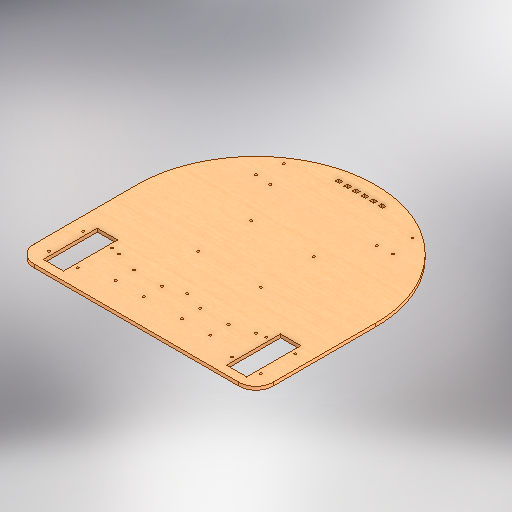
# Autodesk Inventor part: layer1
Saved by Autodesk Inventor 2026 (Build 300175050, 175E)
## iProperties
Created: 2025-06-04
Part Number: layer1
Material: Generic
Document SubType Name: Modeling
Designer: satom
Density: 1 g/cm^3
Appearance: Cherry - Natural Low Gloss
Author: satom
Autodesk Inventor part; units mm, degrees
ref_plane "YZ Plane" through (0, 0, 0) normal (1, 0, 0) x (0, 1, 0)
ref_plane "XZ Plane" through (0, 0, 0) normal (0, 1, 0) x (-1, 0, 0)
ref_plane "XY Plane" through (0, 0, 0) normal (0, 0, 1) x (1, 0, 0)
sketch "Sketch1" plane through (0, 0, 0) normal (0, 1, 0) x (-1, 0, 0)
  arc A0 (-177, 0) -> (177, 0) centre (0, 0) ccw
  line L0 (-177, 0) -> (-177, 151.6)
  line L1 (-151.6, 177) -> (151.6, 177)
  line L2 (177, 151.6) -> (177, 0)
  arc A1 (-151.6, 177) -> (-177, 151.6) centre (-151.6, 151.6) ccw
  arc A2 (177, 151.6) -> (151.6, 177) centre (151.6, 151.6) ccw
  point P0 (-177, 177)
  point P1 (177, 177)
  dimension "d0" = 354
  dimension "d98" = 177
  dimension "d99" = 177
  dimension "d101" = 354
  dimension "d102" = 177
  dimension "d217" = 25.4
  constraints: 6 end point, 6 point on circle, 4 point on line, 4 tangent, 3 centre point, 1 coincident, 1 equal radius, 1 parallel
  measures "d0" diameter of A0
  measures "d98" distance of point (177, 177) L2.end
  measures "d99" distance of L0.start point (-177, 177)
  measures "d101" distance between parallel lines of L0 L2
  measures "d102" distance from line of point (0, 0) L1
  measures "d217" radius of A1
extrude "Extrusion1" add sketch "Sketch1" along normal blind 5
sketch "Sketch8" plane through (0, 5, 0) normal (0, 1, 0) x (1, 0, 0)
  circle A0 centre (101.6, -101.6) radius 1.7
  circle A1 centre (101.6, 101.6) radius 1.7
  circle A2 centre (-101.6, 101.6) radius 1.7
  circle A3 centre (-101.6, -101.6) radius 1.7
  arc A4 (177, 0) -> (-177, 0) centre (0, 0) ccw construction
  line L0 (0, 177) -> (0, -177) construction
  line L1 (-151.6, -177) -> (151.6, -177) construction
  line L2 (-177, 0) -> (-177, -151.6) construction
  line L3 (177, -151.6) -> (177, 0) construction
  line L4 (-177, 0) -> (177, 0) construction
  circle A5 centre (0, -101.6) radius 1.7
  point P0 (0, 0)
  point P1 (-177, -177)
  point P2 (177, -177)
  dimension "d103" = 3.4
  dimension "d104" = 3.4
  dimension "d105" = 3.4
  dimension "d106" = 3.4
  dimension "d115" = 101.6
  dimension "d116" = 101.6
  dimension "d117" = 101.6
  dimension "d118" = 101.6
  dimension "d119" = 101.6
  dimension "d120" = 101.6
  dimension "d121" = 101.6
  dimension "d122" = 101.6
  dimension "d255" = 3.4
  dimension "d256" = 101.6
  constraints: 5 centre point, 4 end point, 2 coincident, 1 horizontal, 1 midpoint, 1 point on circle, 1 point on line
  measures "d103" diameter of A3
  measures "d104" diameter of A2
  measures "d105" diameter of A0
  measures "d106" diameter of A1
  measures "d115" distance from line of L4 A3.centre
  measures "d116" distance from line of L4 A2.centre
  measures "d117" distance from line of L4 A1.centre
  measures "d118" distance from line of L4 A0.centre
  measures "d119" distance from line of A0.centre L0
  measures "d120" distance from line of A3.centre L0
  measures "d121" distance from line of L0 A2.centre
  measures "d122" distance from line of A1.centre L0
  measures "d255" diameter of A5
  measures "d256" distance from line of L4 A5.centre
extrude "Stand-Offs" cut sketch "Sketch8" against normal through all
sketch "Sketch9" plane through (0, 5, 0) normal (0, 1, 0) x (1, 0, 0)
  line L0 (-150.65, -84.3) -> (-150.65, -164.3)
  line L1 (-150.65, -164.3) -> (-120.65, -164.3)
  line L2 (-120.65, -164.3) -> (-120.65, -84.3)
  line L3 (-120.65, -84.3) -> (-150.65, -84.3)
  circle A0 centre (-114.3, -98.9) radius 1.7
  circle A1 centre (-114.3, -149.7) radius 1.7
  circle A2 centre (-157, -149.7) radius 1.7
  circle A3 centre (-157, -98.9) radius 1.7
  arc A4 (177, 0) -> (-177, 0) centre (0, 0) ccw construction
  line L4 (0, 177) -> (0, -177) construction
  line L5 (-151.6, -177) -> (151.6, -177) construction
  line L6 (-120.65, -124.3) -> (-150.65, -124.3) construction
  line L7 (150.65, -164.3) -> (120.65, -164.3)
  line L8 (120.65, -164.3) -> (120.65, -84.3)
  line L9 (120.65, -84.3) -> (150.65, -84.3)
  circle A5 centre (114.3, -98.9) radius 1.7
  circle A6 centre (114.3, -149.7) radius 1.7
  line L10 (150.65, -84.3) -> (150.65, -164.3)
  circle A7 centre (157, -98.9) radius 1.7
  circle A8 centre (157, -149.7) radius 1.7
  line L11 (120.65, -124.3) -> (150.65, -124.3) construction
  line L12 (0, -177) -> (-236.8089, -177) construction
  point P0 (177, -177)
  point P1 (177.1241, 0)
  dimension "d126" = 30
  dimension "d129" = 3.4
  dimension "d130" = 3.4
  dimension "d131" = 3.4
  dimension "d132" = 3.4
  dimension "d133" = 6.35
  dimension "d134" = 6.35
  dimension "d135" = 6.35
  dimension "d136" = 6.35
  dimension "d141" = 120.65
  dimension "d143" = 80
  dimension "d144" = 25.4
  dimension "d145" = 25.4
  dimension "d146" = 25.4
  dimension "d147" = 25.4
  dimension "d236" = 12.7
  constraints: 24 end point, 10 symmetric about line, 8 centre point, 8 coincident, 3 midpoint, 2 parallel, 1 horizontal, 1 perpendicular, 1 point on circle, 4 other
  measures "d126" distance of L2.end L3.end
  measures "d129" diameter of A0
  measures "d130" diameter of A1
  measures "d131" diameter of A2
  measures "d132" diameter of A3
  measures "d133" distance from line of L2 A0.centre
  measures "d134" distance from line of L2 A1.centre
  measures "d135" distance from line of L0 A2.centre
  measures "d136" distance from line of L0 A3.centre
  measures "d141" distance between parallel lines of L4 L2
  measures "d143" distance of L3.end L1.start
  measures "d144" distance from line of L6 A3.centre
  measures "d145" distance from line of L6 A2.centre
  measures "d146" distance from line of L6 A1.centre
  measures "d147" distance from line of L6 A0.centre
  measures "d236" distance between parallel lines of L12 L1
extrude "Wheels" cut sketch "Sketch9" against normal through all
sketch "Sketch10" plane through (0, 5, 0) normal (0, 1, 0) x (1, 0, 0)
  circle A0 centre (-70.11, -137.7493) radius 1.7
  circle A1 centre (-28.3016, -137.7493) radius 1.7
  circle A2 centre (-70.11, -110.8507) radius 1.7
  circle A3 centre (-28.3016, -110.8507) radius 1.7
  arc A4 (177, 0) -> (-177, 0) centre (0, 0) ccw construction
  line L0 (0, 177) -> (0, -177) construction
  line L1 (-151.6, -177) -> (151.6, -177) construction
  line L2 (177, -151.6) -> (177, 0) construction
  line L3 (-177, 0) -> (-177, -151.6) construction
  line L4 (177, 0) -> (-177, 0) construction
  line L5 (-150.65, -84.3) -> (-150.65, -164.3) construction
  line L6 (-150.65, -124.3) -> (150.65, -124.3) construction
  line L7 (150.65, -84.3) -> (150.65, -164.3) construction
  line L8 (-120.65, -84.3) -> (-120.65, -164.3) construction
  circle A5 centre (70.11, -137.7493) radius 1.7
  circle A6 centre (70.11, -110.8507) radius 1.7
  circle A7 centre (28.3016, -137.7493) radius 1.7
  circle A8 centre (28.3016, -110.8507) radius 1.7
  point P0 (-177, -177)
  point P1 (177, -177)
  dimension "d150" = 3.4
  dimension "d151" = 3.4
  dimension "d152" = 3.4
  dimension "d153" = 3.4
  dimension "d154" = 26.8986
  dimension "d155" = 26.8986
  dimension "d156" = 41.8084
  dimension "d157" = 41.8084
  dimension "d161" = 50.54
  dimension "d162" = 13.4493
  dimension "d163" = 13.4493
  dimension "d166" = 13.4493
  dimension "d167" = 13.4493
  constraints: 8 centre point, 6 end point, 4 symmetric about line, 3 midpoint, 1 horizontal, 1 point on circle, 4 other
  measures "d150" diameter of A2
  measures "d151" diameter of A3
  measures "d152" diameter of A0
  measures "d153" diameter of A1
  measures "d154" distance of A0.centre A2.centre
  measures "d155" distance of A1.centre A3.centre
  measures "d156" distance of A1.centre A0.centre
  measures "d157" distance of A2.centre A3.centre
  measures "d161" distance from line of L8 A0.centre
  measures "d162" distance from line of L6 A2.centre
  measures "d163" distance from line of L6 A0.centre
  measures "d166" distance from line of L6 A1.centre
  measures "d167" distance from line of L6 A3.centre
extrude "Motor Mount" cut sketch "Sketch10" against normal through all
sketch "Sketch11" plane through (0, 5, 0) normal (0, 1, 0) x (1, 0, 0)
  circle A0 centre (-46.25, 39.25) radius 1.7
  circle A1 centre (46.25, 39.25) radius 1.7
  circle A2 centre (46.25, -39.25) radius 1.7
  circle A3 centre (-46.25, -39.25) radius 1.7
  line L0 (-177, 0) -> (-177, -151.6) construction
  arc A4 (177, 0) -> (-177, 0) centre (0, 0) ccw construction
  line L1 (-177, 0) -> (177, 0) construction
  line L2 (0, 177) -> (0, -177) construction
  line L3 (-151.6, -177) -> (151.6, -177) construction
  point P0 (-177, -177)
  point P1 (177, -177)
  dimension "d170" = 3.4
  dimension "d171" = 3.4
  dimension "d172" = 3.4
  dimension "d173" = 3.4
  dimension "d174" = 92.5
  dimension "d175" = 92.5
  dimension "d176" = 78.5
  dimension "d177" = 78.5
  dimension "d183" = 46.25
  dimension "d184" = 39.25
  dimension "d185" = 39.25
  dimension "d186" = 46.25
  dimension "d235" = 46.25
  constraints: 4 centre point, 4 end point, 1 horizontal, 1 midpoint, 1 point on circle
  measures "d170" diameter of A0
  measures "d171" diameter of A1
  measures "d172" diameter of A2
  measures "d173" diameter of A3
  measures "d174" distance of A1.centre A0.centre
  measures "d175" distance of A3.centre A2.centre
  measures "d176" distance of A3.centre A0.centre
  measures "d177" distance of A2.centre A1.centre
  measures "d183" distance from line of L2 A3.centre
  measures "d184" distance from line of L1 A0.centre
  measures "d185" distance from line of L1 A1.centre
  measures "d186" distance from line of L2 A0.centre
  measures "d235" distance from line of L2 A1.centre
extrude "PCB" cut sketch "Sketch11" against normal through all
sketch "Sketch12" plane through (0, 5, 0) normal (0, 1, 0) x (1, 0, 0)
  circle A0 centre (95.25, 136.36) radius 1.7
  circle A1 centre (78.74, 99.9262) radius 1.7
  line L0 (-177, 0) -> (-177, -151.6) construction
  line L1 (-177, 0) -> (177, 0) construction
  arc A2 (177, 0) -> (-177, 0) centre (0, 0) ccw construction
  line L2 (78.74, 99.9262) -> (95.25, 136.36) construction
  circle A3 centre (-78.74, 99.9262) radius 1.7
  circle A4 centre (-95.25, 136.36) radius 1.7
  line L3 (0, 177) -> (0, 0) construction
  line L4 (115.2165, 177) -> (-115.2165, 177) construction
  circle A5 centre (101.6, 101.6) radius 1.7 construction
  circle A6 centre (-101.6, 101.6) radius 1.7 construction
  point P0 (-177, -177)
  dimension "d190" = 3.4
  dimension "d191" = 3.4
  dimension "d240" = 40
  dimension "d243" = 95.25
  dimension "d244" = 40
  dimension "d245" = 3.4
  dimension "d246" = 3.4
  dimension "d247" = 40.64
  dimension "d248" = 6.35
  dimension "d249" = 95.25
  dimension "d250" = 6.35
  dimension "d251" = 22.86
  dimension "d252" = 22.86
  dimension "d253" = 40.64
  dimension "d254" = 34.76
  constraints: 8 end point, 4 centre point, 3 coincident, 2 horizontal, 1 midpoint, 1 perpendicular, 1 point on circle
  measures "d190" diameter of A0
  measures "d191" diameter of A1
  measures "d240" distance of L2.start L2.end
  measures "d243" distance from line of L3 A4.centre
  measures "d244" distance of A4.centre A3.centre
  measures "d245" diameter of A3
  measures "d246" diameter of A4
  measures "d247" distance from line of A0.centre L4
  measures "d248" horizontal distance of A0.centre A5.centre
  measures "d249" distance from line of L3 A0.centre
  measures "d250" horizontal distance of A4.centre A6.centre
  measures "d251" horizontal distance of A1.centre A5.centre
  measures "d252" horizontal distance of A6.centre A3.centre
  measures "d253" distance from line of L4 A4.centre
  measures "d254" vertical distance of A5.centre A0.centre
extrude "Ball Caster" cut sketch "Sketch12" against normal through all
sketch "Sketch13" plane through (0, 5, 0) normal (0, 1, 0) x (1, 0, 0)
  line L0 (-34.925, 157.4) -> (-28.575, 157.4)
  line L1 (-28.575, 157.4) -> (-28.575, 152.4)
  line L2 (-28.575, 152.4) -> (-34.925, 152.4)
  line L3 (-34.925, 152.4) -> (-34.925, 157.4)
  line L4 (-22.225, 157.4) -> (-15.875, 157.4)
  line L5 (-15.875, 157.4) -> (-15.875, 152.4)
  line L6 (-15.875, 152.4) -> (-22.225, 152.4)
  line L7 (-22.225, 152.4) -> (-22.225, 157.4)
  line L8 (-9.525, 157.4) -> (-3.175, 157.4)
  line L9 (-3.175, 157.4) -> (-3.175, 152.4)
  line L10 (-3.175, 152.4) -> (-9.525, 152.4)
  line L11 (-9.525, 152.4) -> (-9.525, 157.4)
  line L12 (3.175, 157.4) -> (9.525, 157.4)
  line L13 (9.525, 157.4) -> (9.525, 152.4)
  line L14 (9.525, 152.4) -> (3.175, 152.4)
  line L15 (3.175, 152.4) -> (3.175, 157.4)
  line L16 (15.875, 157.4) -> (22.225, 157.4)
  line L17 (22.225, 157.4) -> (22.225, 152.4)
  line L18 (22.225, 152.4) -> (15.875, 152.4)
  line L19 (15.875, 152.4) -> (15.875, 157.4)
  line L20 (28.575, 157.4) -> (34.925, 157.4)
  line L21 (34.925, 157.4) -> (34.925, 152.4)
  line L22 (34.925, 152.4) -> (28.575, 152.4)
  line L23 (28.575, 152.4) -> (28.575, 157.4)
  arc A0 (177, 0) -> (-177, 0) centre (0, 0) ccw construction
  line L24 (0, 177) -> (0, -177) construction
  line L25 (-151.6, -177) -> (151.6, -177) construction
  line L26 (177, -151.6) -> (177, 0) construction
  line L27 (-177, 0) -> (-177, -151.6) construction
  line L28 (177, 0) -> (-177, 0) construction
  point P0 (-177, -177)
  point P1 (177, -177)
  dimension "d204" = 5
  dimension "d205" = 6.35
  dimension "d208" = 12.7
  dimension "d213" = 152.4
  dimension "d214" = 3.175
  constraints: 52 end point, 3 horizontal, 2 parallel, 1 collinear, 1 midpoint, 1 perpendicular, 1 point on circle, 39 other
  measures "d204" distance of L2.end L0.start
  measures "d205" distance of L0.start L0.end
  measures "d208" distance of L0.start L4.start
  measures "d213" distance between parallel lines of L28 L2
  measures "d214" distance between parallel lines of L24 L15
extrude "Switch" cut sketch "Sketch13" against normal through all
equation "\"d98\" = 0.5 * d0"
equation "\"d99\" = d98"
equation "\"d101\" = d0"
equation "\"d102\" = d99"
equation "\"m3_heat_set_insert\" = 4"
equation "\"m3_clearance\" = 3.4"
equation "\"m3_heat_set_depth\" = 7"
equation "\"hardboard_thickness\" = 5"
equation "\"robot_diameter\" = 354"
equation "\"motor_centerline_height\" = 13"
body "Solid1"
